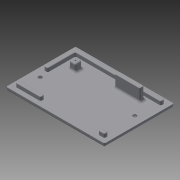
# Autodesk Inventor part: cap
Saved by Autodesk Inventor 2014 SP2 (Build 180246200, 246)
## iProperties
Created: 2024-05-21
Part Number: cap
Material: Generic
Document SubType Name: Sheet Metal
Designer: GauchoHP
Density: 1 g/cm^3
Sheet Metal Rule: Default_mm
Appearance: Default
Author: GauchoHP
Autodesk Inventor part; units mm, degrees
ref_plane "YZ Plane" through (0, 0, 0) normal (1, 0, 0) x (0, 1, 0)
ref_plane "XZ Plane" through (0, 0, 0) normal (0, 1, 0) x (-1, 0, 0)
ref_plane "XY Plane" through (0, 0, 0) normal (0, 0, 1) x (1, 0, 0)
sketch "Sketch1" plane through (0, 0, 0) normal (0, 0, 1) x (1, 0, 0)
  line L0 (-15.2442, 5.8794) -> (60.7558, 5.8794)
  line L1 (61.7558, 4.8794) -> (61.7558, -48.1206)
  line L2 (60.7558, -49.1206) -> (-15.2442, -49.1206)
  line L3 (-16.2442, -48.1206) -> (-16.2442, 4.8794)
  arc A0 (-15.2442, 5.8794) -> (-16.2442, 4.8794) centre (-15.2442, 4.8794) ccw
  arc A1 (61.7558, 4.8794) -> (60.7558, 5.8794) centre (60.7558, 4.8794) ccw
  arc A2 (60.7558, -49.1206) -> (61.7558, -48.1206) centre (60.7558, -48.1206) ccw
  arc A3 (-16.2442, -48.1206) -> (-15.2442, -49.1206) centre (-15.2442, -48.1206) ccw
  point P0 (0, 0)
  point P1 (61.7558, -49.1206)
  point P2 (61.7558, 5.8794)
  point P3 (-16.2442, -49.1206)
  dimension "d0" = 78
  dimension "d1" = 55
  dimension "d2" = 1
  constraints: 8 end point, 8 point on circle, 8 tangent, 6 point on line, 4 centre point, 3 equal radius, 2 parallel, 1 horizontal, 1 perpendicular
  measures "d0" distance of point (61.756, -49.121) point (-16.244, -49.121)
  measures "d1" distance of point (61.756, 5.879) point (61.756, -49.121)
  measures "d2" radius of A0
extrude "Extrusion1" add sketch "Sketch1" along normal blind 3
sketch "Sketch2" plane through (0, 0, 0) normal (0, 0, -1) x (-1, 0, 0)
  line L0 (-61.7558, 4.8794) -> (-61.7558, -48.1206) projected
  line L1 (-60.7558, -49.1206) -> (15.2442, -49.1206) projected
  line L2 (16.2442, -48.1206) -> (16.2442, 4.8794) projected
  circle A0 centre (9.2442, -29.1206) radius 1.5
  circle A1 centre (-54.7558, -18.1206) radius 1.5
  point P0 (0, 0)
  dimension "d5" = 3
  dimension "d6" = 20
  dimension "d7" = 7
  dimension "d8" = 3
  dimension "d9" = 7
  dimension "d10" = 31
  constraints: 2 centre point
  measures "d5" diameter of A0
  measures "d6" distance from line of L1 A0.centre
  measures "d7" distance from line of L2 A0.centre
  measures "d8" diameter of A1
  measures "d9" distance from line of A1.centre L0
  measures "d10" distance from line of L1 A1.centre
extrude "Extrusion2" cut sketch "Sketch2" against normal blind 3
sketch "Sketch3" plane through (0, 0, 3) normal (0, 0, 1) x (1, 0, 0)
  line L0 (60.7558, 5.8794) -> (-15.2442, 5.8794) projected
  line L1 (-16.2442, 4.8794) -> (-16.2442, -48.1206) projected
  line L2 (-12.5442, 2.1794) -> (58.0558, 2.1794)
  line L3 (58.0558, 2.1794) -> (58.0558, -0.8206)
  line L4 (58.0558, -0.8206) -> (-12.5442, -0.8206)
  line L5 (-12.5442, -0.8206) -> (-12.5442, 2.1794)
  line L6 (-15.2442, -49.1206) -> (60.7558, -49.1206) projected
  line L7 (61.7558, -48.1206) -> (61.7558, 4.8794) projected
  line L8 (58.0558, -45.4206) -> (53.0558, -45.4206)
  line L9 (53.0558, -45.4206) -> (53.0558, -42.4206)
  line L10 (53.0558, -42.4206) -> (58.0558, -42.4206)
  line L11 (58.0558, -42.4206) -> (58.0558, -45.4206)
  line L12 (-12.5442, -45.4206) -> (7.4558, -45.4206)
  line L13 (7.4558, -45.4206) -> (7.4558, -42.4206)
  line L14 (7.4558, -42.4206) -> (-12.5442, -42.4206)
  line L15 (-12.5442, -42.4206) -> (-12.5442, -45.4206)
  line L16 (-12.5442, -0.8206) -> (-9.5442, -0.8206)
  line L17 (-9.5442, -0.8206) -> (-9.5442, -22.8206)
  line L18 (-9.5442, -22.8206) -> (-12.5442, -22.8206)
  line L19 (-12.5442, -22.8206) -> (-12.5442, -0.8206)
  point P0 (0, 0)
  dimension "d14" = 3
  dimension "d15" = 3.7
  dimension "d16" = 3.7
  dimension "d19" = 5
  dimension "d20" = 3
  dimension "d21" = 3.7
  dimension "d22" = 3.7
  dimension "d23" = 3.7
  dimension "d24" = 3.7
  dimension "d25" = 20
  dimension "d26" = 3
  dimension "d27" = 22
  dimension "d28" = 28.7
  constraints: 32 end point, 8 parallel, 4 horizontal, 4 perpendicular
  measures "d14" distance of L2.end L3.end
  measures "d15" distance between parallel lines of L0 L2
  measures "d16" distance between parallel lines of L1 L5
  measures "d19" distance of L9.end L10.end
  measures "d20" distance of L8.end L9.end
  measures "d21" distance between parallel lines of L6 L8
  measures "d22" distance between parallel lines of L7 L11
  measures "d23" distance between parallel lines of L7 L3
  measures "d24" distance between parallel lines of L1 L15
  measures "d25" distance of L12.start L12.end
  measures "d26" distance of L17.end L18.end
  measures "d27" distance of L16.end L17.end
  measures "d28" distance between parallel lines of L18 L0
extrude "Extrusion3" add sketch "Sketch3" along normal blind 3
sketch "Sketch4" plane through (0, 0, 3) normal (0, 0, 1) x (1, 0, 0)
  line L0 (60.7558, 5.8794) -> (-15.2442, 5.8794) projected
  line L1 (61.7558, -48.1206) -> (61.7558, 4.8794) projected
  line L2 (47.7558, -7.1206) -> (27.7558, -7.1206)
  line L3 (27.7558, -7.1206) -> (27.7558, -3.6206)
  line L4 (27.7558, -3.6206) -> (47.7558, -3.6206)
  line L5 (47.7558, -3.6206) -> (47.7558, -7.1206)
  line L6 (-16.2442, 4.8794) -> (-16.2442, -48.1206) projected
  line L7 (1.7558, -12.1206) -> (-3.2442, -12.1206)
  line L8 (-3.2442, -12.1206) -> (-3.2442, -7.1206)
  line L9 (-3.2442, -7.1206) -> (1.7558, -7.1206)
  line L10 (1.7558, -7.1206) -> (1.7558, -12.1206)
  line L11 (-0.2442, -9.1206) -> (-1.2442, -9.1206)
  line L12 (-1.2442, -9.1206) -> (-1.2442, -10.1206)
  line L13 (-1.2442, -10.1206) -> (-0.2442, -10.1206)
  line L14 (-0.2442, -10.1206) -> (-0.2442, -9.1206)
  point P0 (0, 0)
  dimension "d30" = 3.5
  dimension "d33" = 9.5
  dimension "d34" = 13
  dimension "d35" = 20
  dimension "d36" = 14
  dimension "d44" = 2
  dimension "d45" = 5
  dimension "d47" = 5
  dimension "d48" = 13
  dimension "d49" = 13
  constraints: 24 end point, 6 parallel, 3 perpendicular, 2 horizontal, 3 other
  measures "d30" distance of L4.end L2.start
  measures "d33" distance between parallel lines of L4 L0
  measures "d34" distance between parallel lines of L0 L2
  measures "d35" distance of L2.start L2.end
  measures "d36" distance between parallel lines of L1 L5
  measures "d44" distance between parallel lines of L9 L11
  measures "d45" distance of L9.end L7.start
  measures "d47" distance of L7.start L8.start
  measures "d48" distance between parallel lines of L6 L8
  measures "d49" distance between parallel lines of L0 L9
extrude "Extrusion4" add sketch "Sketch4" along normal blind 10
sketch "Sketch6" plane through (0, 0, 13) normal (0, 0, 1) x (1, 0, 0)
  line L0 (-0.2442, -9.1206) -> (-0.2442, -10.1206) projected
  line L1 (-0.2442, -10.1206) -> (-1.2442, -10.1206) projected
  line L2 (-1.2442, -10.1206) -> (-1.2442, -9.1206) projected
  line L3 (-1.2442, -9.1206) -> (-0.2442, -9.1206) projected
  line L4 (-3.2442, -12.1206) -> (1.7558, -12.1206) projected
  line L5 (1.7558, -12.1206) -> (1.7558, -7.1206) projected
  line L6 (1.7558, -7.1206) -> (-3.2442, -7.1206) projected
  line L7 (-3.2442, -7.1206) -> (-3.2442, -12.1206) projected
  point P0 (0, 0)
extrude "Extrusion6" cut sketch "Sketch6" against normal blind 4
fillet "Fillet1" radius 1 14 edges at (58.0558, 2.1794, 4.5) (-12.5442, 2.1794, 4.5) (-12.5442, -22.8206, 4.5) (-9.5442, -22.8206, 4.5) (-9.5442, -0.8206, 4.5) (58.0558, -0.8206, 4.5) (47.7558, -3.6206, 8) (47.7558, -7.1206, 8) (27.7558, -7.1206, 8) (27.7558, -3.6206, 8) (-3.2442, -12.1206, 6) (1.7558, -12.1206, 6) (-3.2442, -7.1206, 6) (1.7558, -7.1206, 6)
fillet "Fillet2" radius 0.5 20 edges at (-9.2513, -1.1135, 6) (24.2558, -0.8206, 6) (-9.8371, -22.5277, 6) (-11.0442, -22.8206, 6) (-12.2513, -22.5277, 6) (-12.5442, -10.3206, 6) (-12.2513, 1.8865, 6) (22.7558, 2.1794, 6) (57.7629, 1.8865, 6) (58.0558, 0.6794, 6) (57.7629, -0.5277, 6) (-9.5442, -11.8206, 6) (47.4629, -6.8277, 13) (47.7558, -5.3706, 13) (47.4629, -3.9135, 13) (37.7558, -3.6206, 13) (28.0487, -3.9135, 13) (27.7558, -5.3706, 13) (28.0487, -6.8277, 13) (37.7558, -7.1206, 13)
fillet "Fillet3" radius 1 8 edges at (53.0558, -42.4206, 4.5) (53.0558, -45.4206, 4.5) (58.0558, -45.4206, 4.5) (58.0558, -42.4206, 4.5) (7.4558, -45.4206, 4.5) (7.4558, -42.4206, 4.5) (-12.5442, -45.4206, 4.5) (-12.5442, -42.4206, 4.5)
fillet "Fillet4" radius 0.5 16 edges at (7.1629, -45.1277, 6) (7.4558, -43.9206, 6) (7.1629, -42.7135, 6) (-2.5442, -42.4206, 6) (-12.2513, -42.7135, 6) (-12.5442, -43.9206, 6) (-12.2513, -45.1277, 6) (-2.5442, -45.4206, 6) (53.0558, -43.9206, 6) (53.3487, -42.7135, 6) (55.5558, -42.4206, 6) (57.7629, -42.7135, 6) (58.0558, -43.9206, 6) (57.7629, -45.1277, 6) (55.5558, -45.4206, 6) (53.3487, -45.1277, 6)
fillet "Fillet5" radius 2 15 edges at (28.0487, -6.8277, 3) (27.7558, -5.3706, 3) (28.0487, -3.9135, 3) (47.4629, -6.8277, 3) (47.7558, -5.3706, 3) (47.4629, -3.9135, 3) (37.7558, -7.1206, 3) (-2.9513, -11.8277, 3) (-3.2442, -9.6206, 3) (-2.9513, -7.4135, 3) (-0.7442, -7.1206, 3) (1.4629, -7.4135, 3) (1.7558, -9.6206, 3) (1.4629, -11.8277, 3) (-0.7442, -12.1206, 3)
fillet "Fillet6" radius 0.5 20 edges at (28.7558, -6.9741, 12.8536) (28.4023, -6.4741, 13) (27.9023, -6.1206, 12.8536) (28.2558, -5.3706, 13) (27.9023, -4.6206, 12.8536) (46.7558, -6.9741, 12.8536) (37.7558, -6.6206, 13) (28.4023, -4.267, 13) (28.7558, -3.767, 12.8536) (47.6094, -6.1206, 12.8536) (47.1094, -6.4741, 13) (37.7558, -4.1206, 13) (46.7558, -3.767, 12.8536) (47.6094, -4.6206, 12.8536) (47.2558, -5.3706, 13) (47.1094, -4.267, 13) (-0.2442, -9.1206, 6) (-1.2442, -9.1206, 6) (-0.2442, -10.1206, 6) (-1.2442, -10.1206, 6)
chamfer "Chamfer1" distance 2.5 angle 45 2 edges at (-7.7442, -29.1206, 0) (56.2558, -18.1206, 0)
chamfer "Chamfer2" distance 1 angle 45 8 edges at (22.7558, 5.8794, 0) (61.4629, 5.5865, 0) (61.7558, -21.6206, 0) (61.4629, -48.8277, 0) (22.7558, -49.1206, 0) (-15.9513, -48.8277, 0) (-16.2442, -21.6206, 0) (-15.9513, 5.5865, 0)
fillet "Fillet7" radius 1 8 edges at (61.4629, -48.8277, 0.9999) (22.7558, -49.1206, 0.9999) (-15.9513, -48.8277, 0.9999) (-16.2442, -21.6206, 0.9999) (-15.9513, 5.5865, 0.9999) (22.7558, 5.8794, 0.9999) (61.4629, 5.5865, 0.9999) (61.7558, -21.6206, 0.9999)
fillet "Fillet9" radius 1 8 edges at (-2.9513, -11.8277, 9) (-3.2442, -9.6206, 9) (-2.9513, -7.4135, 9) (-0.7442, -7.1206, 9) (1.4629, -7.4135, 9) (1.7558, -9.6206, 9) (1.4629, -11.8277, 9) (-0.7442, -12.1206, 9)
equation "\"BendRadius\" = Thickness"
equation "\"BendReliefWidth\" = Thickness"
equation "\"BendReliefDepth\" = 0.5 * Thickness"
equation "\"CornerReliefSize\" = 4 * Thickness"
equation "\"MinimumRemnant\" = 2 * Thickness"
equation "\"TransitionRadius\" = BendRadius"
equation "\"JacobiRadiusSize\" = BendRadius"
equation "\"GapSize\" = Thickness"
equation "\"Thickness\" = 0.5"
body "Solid1"
